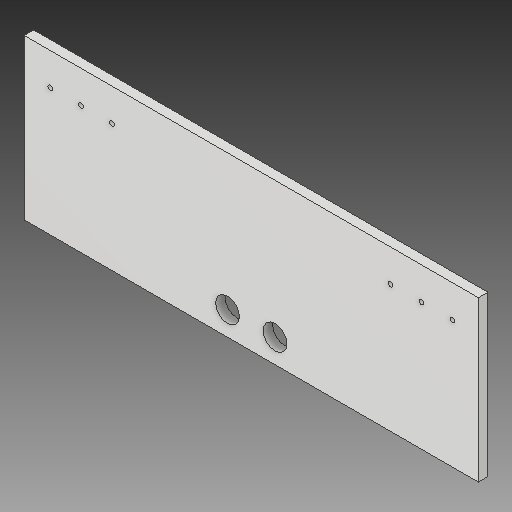
# Autodesk Inventor part: TC005b
Saved by Autodesk Inventor 2017 SP1 (Build 210196100, 196)
## iProperties
Created: 2018-01-07
Part Number: TC005b
Material: ABS Plastic
Document SubType Name: Modeling
Designer: Zach
Density: 1.06 g/cm^3
Appearance: CR White
Mass: 839.567 g
Surface Area: 1738.42 cm^2
Volume: 792.044 cm^3
Author: Zach
Autodesk Inventor part; units mm, degrees
ref_plane "YZ Plane" through (0, 0, 0) normal (1, 0, 0) x (0, 1, 0)
ref_plane "XZ Plane" through (0, 0, 0) normal (0, 1, 0) x (-1, 0, 0)
ref_plane "XY Plane" through (0, 0, 0) normal (0, 0, 1) x (1, 0, 0)
sketch "Sketch1" plane through (0, 0, 0) normal (0, 0, 1) x (1, 0, 0)
  line L0 (0, 0) -> (478, 0)
  line L1 (478, 0) -> (478, 168)
  line L2 (478, 168) -> (0, 168)
  line L3 (0, 168) -> (0, 0)
  dimension "d0" = 478
  dimension "d1" = 168
  constraints: 8 end point, 2 parallel, 1 horizontal, 1 perpendicular
  measures "d0" distance of L2.end L1.end
  measures "d1" distance of L1.end L0.end
extrude "Extrusion1" add sketch "Sketch1" along normal blind 10
sketch "Sketch2" plane through (0, 0, 10) normal (0, 0, 1) x (1, 0, 0)
  circle A0 centre (27.5, 134) radius 2.5
  circle A1 centre (92.5, 134) radius 2.5
  line L0 (478, 168) -> (0, 168) projected
  line L1 (0, 168) -> (0, 0) projected
  circle A2 centre (385.5, 134) radius 2.5
  circle A3 centre (450.5, 134) radius 2.5
  line L2 (478, 0) -> (478, 168) projected
  line L3 (27.5, 134) -> (92.5, 134) construction
  line L4 (385.5, 134) -> (450.5, 134) construction
  circle A4 centre (60, 134) radius 2.5
  circle A5 centre (418, 134) radius 2.5
  dimension "d5" = 5
  dimension "d6" = 5
  dimension "d7" = 65
  dimension "d8" = 34
  dimension "d9" = 27.5
  dimension "d10" = 5
  dimension "d11" = 5
  dimension "d12" = 65
  dimension "d13" = 27.5
  dimension "d28" = 5
  dimension "d29" = 5
  constraints: 6 centre point, 4 end point, 3 horizontal alignment, 2 horizontal, 2 midpoint
  measures "d5" diameter of A0
  measures "d6" diameter of A1
  measures "d7" distance of L3.start L3.end
  measures "d8" distance from line of L0 L3.start
  measures "d9" distance from line of L1 L3.start
  measures "d10" diameter of A2
  measures "d11" diameter of A3
  measures "d12" distance of L4.start L4.end
  measures "d13" distance from line of L2 L4.end
  measures "d28" diameter of A4
  measures "d29" diameter of A5
extrude "Extrusion2" cut sketch "Sketch2" against normal through all
sketch "Sketch3" plane through (0, 0, 10) normal (0, 0, 1) x (1, 0, 0)
  line L0 (189, 85) -> (289, 85)
  line L1 (289, 85) -> (289, 15)
  line L2 (289, 15) -> (189, 15)
  line L3 (189, 15) -> (189, 85)
  line L4 (0, 0) -> (478, 0) projected
  point P0 (239, 15)
  point P1 (239, 0)
  dimension "d16" = 100
  dimension "d17" = 70
  dimension "d18" = 15
  constraints: 8 end point, 2 midpoint, 2 parallel, 1 horizontal, 1 perpendicular, 1 vertical alignment
  measures "d16" distance of L1.end L2.end
  measures "d17" distance of L0.end L1.end
  measures "d18" distance between parallel lines of L4 L2
extrude "Extrusion3" [suppressed]
sketch "Sketch6" plane through (289, 15, 10) normal (-1, 0, 0) x (0, 0, 1)
  line L0 (0, 70) -> (0, 0) projected
  line L1 (0, 70) -> (-7, 70) projected
  line L2 (-7, 70) -> (-7, 0) construction
  line L3 (0, 0) -> (-7, 0) projected
  line L4 (-7, 70) -> (8, 70) construction
  line L5 (8, 70) -> (8, 25) construction
  line L6 (8, 25) -> (-7, 25) construction
  line L7 (-7, 25) -> (-7, 70)
  line L8 (8, 25) -> (18, 25)
  line L9 (0, -15) -> (0, 153) projected
  arc A0 (18, 25) -> (0, 100) centre (-131.9551, 28.6708) ccw
  line L10 (0, 100) -> (0, 70)
  line L11 (0, 70) -> (8, 70)
  line L12 (8, 70) -> (8, 25)
  point P0 (-10, -15)
  dimension "d33" = 15
  dimension "d34" = 25
  dimension "d35" = 10
  dimension "d36" = 150
  dimension "d37" = 30
  constraints: 16 end point, 3 horizontal, 2 parallel, 2 perpendicular, 2 point on circle, 1 centre point, 1 point on line, 1 vertical
  measures "d33" distance of L5.end L6.end
  measures "d34" distance between parallel lines of L3 L6
  measures "d35" distance of L5.end L8.end
  measures "d36" radius of A0
  measures "d37" distance from line of L10.start L4
extrude "Extrusion6" [suppressed]
sketch "Sketch7" plane through (189, 15, 10) normal (-1, 0, 0) x (0, 0, 1)
  arc A0 (18, 25) -> (0, 100) centre (-131.9551, 28.6708) ccw projected
  line L0 (18, 25) -> (0, 25)
  line L1 (0, 153) -> (0, -15) projected
  line L2 (0, 25) -> (0, 100)
  point P0 (-10, -15)
  constraints: 4 end point, 1 horizontal, 1 perpendicular, 1 point on line
extrude "Extrusion7" [suppressed]
sketch "Sketch8" plane through (289, 15, 10) normal (1, 0, 0) x (0, 0, -1)
  arc A0 (0, 100) -> (-18, 25) centre (131.9551, 28.6708) ccw projected
  line L0 (0, 25) -> (0, 100) projected
  line L1 (0, 25) -> (-18, 25) projected
  point P0 (10, -15)
extrude "Extrusion8" [suppressed]
sketch "Sketch9" plane through (0, 0, 10) normal (0, 0, 1) x (1, 0, 0)
  line L0 (214, 25) -> (264, 25) construction
  circle A0 centre (264, 25) radius 12.5
  circle A1 centre (214, 25) radius 12.5
  line L1 (0, 0) -> (478, 0) construction
  point P0 (239, 25)
  point P1 (239, 0)
  dimension "d45" = 50
  dimension "d46" = 25
  dimension "d47" = 25
  dimension "d48" = 25
  constraints: 2 centre point, 2 coincident, 2 end point, 2 midpoint, 1 horizontal, 1 vertical alignment
  measures "d45" distance of L0.start L0.end
  measures "d46" diameter of A0
  measures "d47" diameter of A1
  measures "d48" distance between parallel lines of L1 L0
extrude "Extrusion9" cut sketch "Sketch9" against normal through all
body "Solid1"
